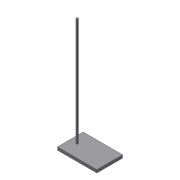
# Autodesk Inventor part: teststand
Saved by Autodesk Inventor 2017 (Build 210142000, 142)
## iProperties
Created: 2021-08-28
Part Number: teststand
Material: Generic
Document SubType Name: Modeling
Designer: jwoods
Density: 1 g/cm^3
Appearance: Default
Author: jwoods
Autodesk Inventor part; units mm, degrees
ref_plane "YZ Plane" through (0, 0, 0) normal (1, 0, 0) x (0, 1, 0)
ref_plane "XZ Plane" through (0, 0, 0) normal (0, 1, 0) x (-1, 0, 0)
ref_plane "XY Plane" through (0, 0, 0) normal (0, 0, 1) x (1, 0, 0)
sketch "Sketch1" plane through (0, 0, 0) normal (0, 1, 0) x (-1, 0, 0)
  line L0 (159.7591, 78.536) -> (-52.9659, 78.536)
  line L1 (-52.9659, 78.536) -> (-52.9659, -60.184)
  line L2 (-52.9659, -60.184) -> (159.7591, -60.184)
  line L3 (159.7591, -60.184) -> (159.7591, 78.536)
  point P0 (0, 0)
  dimension "d0" = 138.72
  dimension "d1" = 212.725
  constraints: 8 end point, 2 parallel, 1 horizontal, 1 perpendicular
  measures "d0" distance of L0.end L1.end
  measures "d1" distance of L1.end L2.end
extrude "Extrusion1" add sketch "Sketch1" along normal blind 16
sketch "Sketch2" plane through (0, 16, 0) normal (0, 1, 0) x (1, 0, 0)
  line L0 (-159.7591, -78.536) -> (52.9659, -78.536) projected
  line L1 (52.9659, -78.536) -> (52.9659, 60.184) projected
  line L2 (52.9659, 60.184) -> (-159.7591, 60.184) projected
  line L3 (-159.7591, 60.184) -> (-159.7591, -78.536) projected
  line L4 (-159.7591, 60.184) -> (-159.7591, -78.536) projected
  line L5 (-159.7591, -9.176) -> (52.9659, -9.176)
  line L6 (52.9659, -78.536) -> (52.9659, 60.184) projected
  circle A0 centre (-122.3691, -9.176) radius 5.89
  line L7 (-122.3691, -9.176) -> (-128.2591, -9.176)
  point P0 (0, 0)
  dimension "d4" = 11.78
  dimension "d5" = 31.5
  constraints: 4 end point, 2 midpoint, 2 point on line, 1 horizontal alignment, 2 other
  measures "d5" distance of L5.start L7.end
extrude "Extrusion2" add sketch "Sketch2" along normal blind 584.2 contours A0 L5 | L5 A0
sketch "Sketch3" plane through (52.9659, 0, 78.536) normal (1, 0, 0) x (0, 0, -1)
  line L0 (0, 0) -> (138.72, 0) projected
  line L1 (138.72, 0) -> (138.72, 16) projected
  line L2 (0, 16) -> (138.72, 16) projected
  line L3 (0, 0) -> (0, 16) projected
  line L4 (0, 8) -> (138.72, 8)
  circle A0 centre (69.36, 8) radius 3.5
  point P0 (78.536, 0)
  dimension "d8" = 7
  constraints: 3 midpoint, 2 end point, 1 centre point
  measures "d8" diameter of A0
extrude "Extrusion3" cut sketch "Sketch3" against normal blind 0.25 contours A0 L4 | L4 A0
body "Solid1"
